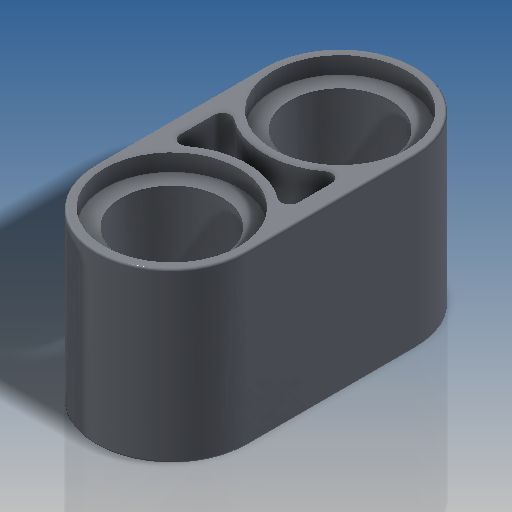
# Autodesk Inventor part: 43857-LtBluishGray
Saved by Autodesk Inventor 2018.3 (Build 223284000, 284)
## iProperties
Created: 2012-03-21
Part Number: 43857-LtBluishGray
Document SubType Name: Modeling
Designer: D. Kohfeld
Density: 1.06 g/cm^3
Material: ABS Plastic
Mass: 0.424026 g
Surface Area: 7.86496 cm^2
Volume: 0.400024 cm^3
Appearance: LtBluishGray
Author: D. Kohfeld
Autodesk Inventor part; units mm, degrees
ref_plane "YZ Plane" through (0, 0, 0) normal (1, 0, 0) x (0, 1, 0)
ref_plane "XZ Plane" through (0, 0, 0) normal (0, 1, 0) x (-1, 0, 0)
ref_plane "XY Plane" through (0, 0, 0) normal (0, 0, 1) x (1, 0, 0)
sketch "Sketch1" plane through (0, 0, 0) normal (0, 0, 1) x (1, 0, 0)
  line L0 (3.6, 0) -> (3.6, 8)
  line L1 (-3.6, 8) -> (-3.6, 0)
  arc A0 (3.6, 8) -> (-3.6, 8) centre (0, 8) ccw
  circle A1 centre (0, 8) radius 2.4
  circle A2 centre (0, 8) radius 3.2
  circle A3 centre (0, 0) radius 3.2
  circle A4 centre (0, 0) radius 2.4
  line L2 (0, 0) -> (0, 8) construction
  line L3 (-2.8, 5.7373) -> (-2.8, 2.2627)
  line L4 (2.8, 5.7373) -> (2.8, 2.2627)
  arc A5 (-2.8, 5.7373) -> (2.8, 5.7373) centre (0, 8) ccw
  arc A6 (2.8, 2.2627) -> (-2.8, 2.2627) centre (0, 0) ccw
  arc A7 (-3.6, 0) -> (3.6, 0) centre (0, 0) ccw
  line L5 (0, 0) -> (0, -8) construction
  dimension "d8" = 4.8
  dimension "d9" = 6.4
  dimension "d32" = 7.2
  dimension "d34" = 8
  dimension "d36" = 0.8
  constraints: 12 end point, 8 centre point, 8 point on circle, 7 coincident, 4 equal radius, 4 tangent, 3 parallel, 2 equal length, 2 vertical
  measures "d8" diameter of A1
  measures "d9" diameter of A2
  measures "d32" diameter of A0
  measures "d34" distance of L2.start L2.end
  measures "d36" distance between parallel lines of L1 L3
extrude "Extrusion1" add sketch "Sketch1" along normal mid plane 8 contours A7 L1 A0 L0 | A2 | A3 | A5 L4 A6 L3
sketch "Sketch6" plane through (0, 0, 4) normal (0, 0, 1) x (1, 0, 0)
  circle A0 centre (0, 0) radius 2.4 projected
  circle A1 centre (0, 8) radius 2.4 projected
  circle A2 centre (0, 0) radius 3.2 projected
  circle A3 centre (0, 8) radius 3.2 projected
  arc A4 (2.8, 2.2627) -> (-2.8, 2.2627) centre (0, 0) ccw projected
  line L0 (-2.8, 5.7373) -> (-2.8, 2.2627) projected
  arc A5 (-2.8, 5.7373) -> (2.8, 5.7373) centre (0, 8) ccw projected
  line L1 (2.8, 5.7373) -> (2.8, 2.2627) projected
extrude "Extrusion7" cut sketch "Sketch6" against normal blind 0.8 contours A2 | A3
extrude "Extrusion8" cut sketch "Sketch6" against normal blind 3.1 contours A4 L0 A5 L1
mirror "Mirror1" about plane through (0, 0, 0) normal (0, 0, 1) of "Extrusion7", "Extrusion8"
fillet "Fillet1" radius 0.1 6 edges at (0, 11.6, 4) (3.6, 4, 4) (-3.6, 4, 4) (0, 11.6, -4) (-3.6, 4, -4) (3.6, 4, -4)
fillet "Fillet1" radius 0.4 8 edges at (-2.8, 2.2627, 2.45) (-2.8, 5.7373, 2.45) (2.8, 2.2627, 2.45) (2.8, 5.7373, 2.45) (2.8, 5.7373, -2.45) (2.8, 2.2627, -2.45) (-2.8, 2.2627, -2.45) (-2.8, 5.7373, -2.45)
equation "\"d8\" = tpd"
equation "\"d9\" = tsd"
equation "\"d32\" = tlad"
equation "\"d34\" = lu"
equation "\"d14\" = lu"
equation "\"d41\" = tsl"
equation "\"d45\" = lf"
equation "\"d46\" = tf"
equation "\"tpd\" = 4.8"
equation "\"tsd\" = 6.4"
equation "\"tlad\" = 7.2"
equation "\"lu\" = 8"
equation "\"tsl\" = 0.8"
equation "\"lf\" = 0.1"
equation "\"tf\" = 0.4"
body "Solid1"
